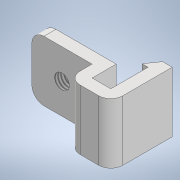
# Autodesk Inventor part: cantoneira
Saved by Autodesk Inventor 2021 (Build 250183000, 183)
## iProperties
Created: 2022-08-18
Part Number: cantoneira
Material: Genérico
Document SubType Name: Modeling
Designer: 21155060
Density: 1 g/cm^3
Appearance: Padrão
Author: 21155060
Autodesk Inventor part; units mm, degrees
ref_plane "YZ Plane" through (0, 0, 0) normal (1, 0, 0) x (0, 1, 0)
ref_plane "XZ Plane" through (0, 0, 0) normal (0, 1, 0) x (-1, 0, 0)
ref_plane "XY Plane" through (0, 0, 0) normal (0, 0, 1) x (1, 0, 0)
sketch "Esboço1" plane through (0, 0, 0) normal (0, 1, 0) x (-1, 0, 0)
  line L0 (0, 0) -> (0, 2)
  line L1 (0, 2) -> (-10, 2)
  line L2 (-10, 2) -> (-10, 4)
  line L3 (-10, 4) -> (-17.1, 4)
  line L4 (-17.1, 4) -> (-17.1, -6.2)
  line L5 (-17.1, -6.2) -> (-15.5004, -6.2)
  line L6 (-15.5004, -6.2) -> (-14.1, -4.2)
  line L7 (-14.1, -4.2) -> (-15.1, -4.2)
  line L8 (-15.1, -4.2) -> (-15.1, 2)
  line L9 (-15.1, 2) -> (-12, 2)
  line L10 (-12, 2) -> (-12, 0)
  line L11 (-12, 0) -> (0, 0)
  line L12 (-12, 0) -> (-11.1591, 0) construction
  line L13 (-10, 0) -> (-10, -4.2)
  line L14 (-10, -4.2) -> (-12, -4.2)
  line L15 (-12, -4.2) -> (-12, 0)
  line L16 (-11.1591, 0) -> (-10, 0) construction
  dimension "d0" = 2
  dimension "d1" = 55
  dimension "d2" = 10
  dimension "d3" = 6.2
  dimension "d4" = 2
  dimension "d5" = 2
  dimension "d6" = 2
  dimension "d7" = 3.1
  dimension "d8" = 1
  dimension "d10" = 2
  dimension "d11" = 2
  dimension "d12" = 12
  dimension "d25" = 2
  constraints: 34 end point, 10 perpendicular, 4 parallel, 2 horizontal, 1 collinear, 1 point on line, 1 vertical
  measures "d0" distance of L0.start L0.end
  measures "d1" angle of L7 L6
  measures "d2" distance of L0.end L1.end
  measures "d3" distance of L7.end L8.end
  measures "d4" distance between parallel lines of L3 L9
  measures "d5" distance between parallel lines of L10 L2
  measures "d6" distance between parallel lines of L4 L8
  measures "d7" distance between parallel lines of L10 L8
  measures "d8" distance of L6.end L7.end
  measures "d10" distance of L1.end L2.end
  measures "d11" distance between parallel lines of L7 L5
  measures "d12" distance of L10.end L0.start
  measures "d25" distance of L13.end L14.end
extrude "Extrusão1" add sketch "Esboço1" along normal blind 10
sketch "Esboço2" plane through (0, 0, 2) normal (0, 0, 1) x (1, 0, 0)
  line L0 (0, 0) -> (0, 10) projected
  line L1 (0, 0) -> (10, 0) projected
  point P0 (5, 5)
  dimension "d15" = 5
  dimension "d16" = 5
  measures "d15" distance from line of L0 point (5, 5)
  measures "d16" distance from line of L1 point (5, 5)
hole "Furo1" at (5, 5, 2) direction (0, 0, -1) diameter 2.459 end through all thread size "M3x0.5" class "6H" standard "ISO Metric profile"
fillet "Arredondamento1" radius 2 5 edges at (17.1, 5, 4) (10, 5, 4) (0, 10, 1) (0, 0, 1) (10, 5, -4.2)
